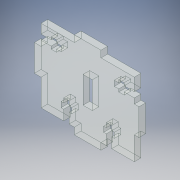
# Autodesk Inventor part: Refuerzo_Conducto
Saved by Autodesk Inventor 2019 (Build 230136000, 136)
## iProperties
Created: 2020-04-06
Part Number: Refuerzo_Conducto
Material: Generic
Document SubType Name: Modeling
Designer: Jurgen
Density: 1 g/cm^3
Appearance: Clear
Author: Jurgen
Autodesk Inventor part; units mm, degrees
ref_plane "YZ Plane" through (0, 0, 0) normal (1, 0, 0) x (0, 1, 0)
ref_plane "XZ Plane" through (0, 0, 0) normal (0, 1, 0) x (-1, 0, 0)
ref_plane "XY Plane" through (0, 0, 0) normal (0, 0, 1) x (1, 0, 0)
sketch "Sketch1" plane through (0, 0, 0) normal (0, 0, 1) x (1, 0, 0)
  line L0 (-35, -27.5) -> (35, -27.5)
  line L1 (35, -27.5) -> (35, 27.5)
  line L2 (35, 27.5) -> (-35, 27.5)
  line L3 (-35, 27.5) -> (-35, -27.5)
  line L4 (-35, -27.5) -> (35, 27.5) construction
  line L5 (35, -27.5) -> (-35, 27.5) construction
  point P0 (0, 0)
  dimension "d0" = 70
  dimension "d1" = 55
  constraints: 12 end point, 2 midpoint, 2 parallel, 1 horizontal, 1 perpendicular
  measures "d0" distance of L2.end L1.end
  measures "d1" distance of L1.end L0.end
extrude "Extrusion1" add sketch "Sketch1" along normal blind 5
sketch "Sketch2" plane through (0, 0, 5) normal (0, 0, 1) x (1, 0, 0)
  line L0 (-35, -27.5) -> (35, -27.5) construction
  line L1 (35, -27.5) -> (35, 27.5) construction
  line L2 (35, 27.5) -> (-35, 27.5) construction
  line L3 (-35, 27.5) -> (-35, -27.5) construction
  line L4 (-10, -27.5) -> (10, -27.5)
  line L5 (10, -27.5) -> (10, -32.5)
  line L6 (10, -32.5) -> (-10, -32.5)
  line L7 (-10, -32.5) -> (-10, -27.5)
  line L8 (-35, -7.5) -> (-40, -7.5)
  line L9 (-40, -7.5) -> (-40, 12.5)
  line L10 (-40, 12.5) -> (-35, 12.5)
  line L11 (-35, 12.5) -> (-35, -7.5)
  line L12 (35, 27.5) -> (-35, 27.5) construction
  line L13 (-10, 27.5) -> (10, 27.5)
  line L14 (10, 27.5) -> (10, 32.5)
  line L15 (10, 32.5) -> (-10, 32.5)
  line L16 (-10, 32.5) -> (-10, 27.5)
  line L17 (35, 18) -> (35, 14) construction
  line L18 (35, 14) -> (20, 14) construction
  line L19 (20, 14) -> (20, 18) construction
  line L20 (20, 18) -> (35, 18) construction
  line L21 (35, 16) -> (20, 16) construction
  line L22 (23.3333, 20) -> (23.3333, 12) construction
  line L23 (23.3333, 12) -> (27.3333, 12) construction
  line L24 (27.3333, 12) -> (27.3333, 20) construction
  line L25 (27.3333, 20) -> (23.3333, 20) construction
  line L26 (23.3333, 20) -> (27.3333, 12) construction
  line L27 (23.3333, 12) -> (27.3333, 20) construction
  line L28 (35, 18) -> (27.3333, 18)
  line L29 (27.3333, 18) -> (27.3333, 20)
  line L30 (27.3333, 20) -> (23.3333, 20)
  line L31 (23.3333, 20) -> (23.3333, 18)
  line L32 (23.3333, 18) -> (20, 18)
  line L33 (20, 18) -> (20, 14)
  line L34 (20, 14) -> (23.3333, 14)
  line L35 (23.3333, 14) -> (23.3333, 12)
  line L36 (23.3333, 12) -> (27.3333, 12)
  line L37 (27.3333, 12) -> (27.3333, 14)
  line L38 (27.3333, 14) -> (35, 14)
  line L39 (35, 14) -> (35, 18)
  line L40 (-35, 16.5) -> (-35, 20.5) construction
  line L41 (-35, 20.5) -> (-20, 20.5) construction
  line L42 (-20, 20.5) -> (-20, 16.5) construction
  line L43 (-20, 16.5) -> (-35, 16.5) construction
  line L44 (-35, 18.5) -> (-20, 18.5) construction
  line L45 (-23.3333, 14.5) -> (-23.3333, 22.5) construction
  line L46 (-23.3333, 22.5) -> (-27.3333, 22.5) construction
  line L47 (-27.3333, 22.5) -> (-27.3333, 14.5) construction
  line L48 (-27.3333, 14.5) -> (-23.3333, 14.5) construction
  line L49 (-23.3333, 14.5) -> (-27.3333, 22.5) construction
  line L50 (-23.3333, 22.5) -> (-27.3333, 14.5) construction
  line L51 (-35, 16.5) -> (-27.3333, 16.5)
  line L52 (-27.3333, 16.5) -> (-27.3333, 14.5)
  line L53 (-27.3333, 14.5) -> (-23.3333, 14.5)
  line L54 (-23.3333, 14.5) -> (-23.3333, 16.5)
  line L55 (-23.3333, 16.5) -> (-20, 16.5)
  line L56 (-20, 16.5) -> (-20, 20.5)
  line L57 (-20, 20.5) -> (-23.3333, 20.5)
  line L58 (-23.3333, 20.5) -> (-23.3333, 22.5)
  line L59 (-23.3333, 22.5) -> (-27.3333, 22.5)
  line L60 (-27.3333, 22.5) -> (-27.3333, 20.5)
  line L61 (-27.3333, 20.5) -> (-35, 20.5)
  line L62 (-35, 20.5) -> (-35, 16.5)
  line L63 (-14, -27.5) -> (-18, -27.5) construction
  line L64 (-18, -27.5) -> (-18, -12.5) construction
  line L65 (-18, -12.5) -> (-14, -12.5) construction
  line L66 (-14, -12.5) -> (-14, -27.5) construction
  line L67 (-16, -27.5) -> (-16, -12.5) construction
  line L68 (-12, -15.8333) -> (-20, -15.8333) construction
  line L69 (-20, -15.8333) -> (-20, -19.8333) construction
  line L70 (-20, -19.8333) -> (-12, -19.8333) construction
  line L71 (-12, -19.8333) -> (-12, -15.8333) construction
  line L72 (-12, -15.8333) -> (-20, -19.8333) construction
  line L73 (-20, -15.8333) -> (-12, -19.8333) construction
  line L74 (-14, -27.5) -> (-14, -19.8333)
  line L75 (-14, -19.8333) -> (-12, -19.8333)
  line L76 (-12, -19.8333) -> (-12, -15.8333)
  line L77 (-12, -15.8333) -> (-14, -15.8333)
  line L78 (-14, -15.8333) -> (-14, -12.5)
  line L79 (-14, -12.5) -> (-18, -12.5)
  line L80 (-18, -12.5) -> (-18, -15.8333)
  line L81 (-18, -15.8333) -> (-20, -15.8333)
  line L82 (-20, -15.8333) -> (-20, -19.8333)
  line L83 (-20, -19.8333) -> (-18, -19.8333)
  line L84 (-18, -19.8333) -> (-18, -27.5)
  line L85 (-18, -27.5) -> (-14, -27.5)
  line L86 (18, -27.5) -> (14, -27.5) construction
  line L87 (14, -27.5) -> (14, -12.5) construction
  line L88 (14, -12.5) -> (18, -12.5) construction
  line L89 (18, -12.5) -> (18, -27.5) construction
  line L90 (16, -27.5) -> (16, -12.5) construction
  line L91 (20, -15.8333) -> (12, -15.8333) construction
  line L92 (12, -15.8333) -> (12, -19.8333) construction
  line L93 (12, -19.8333) -> (20, -19.8333) construction
  line L94 (20, -19.8333) -> (20, -15.8333) construction
  line L95 (20, -15.8333) -> (12, -19.8333) construction
  line L96 (12, -15.8333) -> (20, -19.8333) construction
  line L97 (18, -27.5) -> (18, -19.8333)
  line L98 (18, -19.8333) -> (20, -19.8333)
  line L99 (20, -19.8333) -> (20, -15.8333)
  line L100 (20, -15.8333) -> (18, -15.8333)
  line L101 (18, -15.8333) -> (18, -12.5)
  line L102 (18, -12.5) -> (14, -12.5)
  line L103 (14, -12.5) -> (14, -15.8333)
  line L104 (14, -15.8333) -> (12, -15.8333)
  line L105 (12, -15.8333) -> (12, -19.8333)
  line L106 (12, -19.8333) -> (14, -19.8333)
  line L107 (14, -19.8333) -> (14, -27.5)
  line L108 (14, -27.5) -> (18, -27.5)
  line L109 (35, -27.5) -> (35, 27.5) construction
  line L110 (35, 10) -> (38.5, 10)
  line L111 (38.5, 10) -> (38.5, -10)
  line L112 (38.5, -10) -> (35, -10)
  line L113 (35, -10) -> (35, 10)
  point P0 (0, 0)
  point P1 (25.3333, 16)
  point P2 (-25.3333, 18.5)
  point P3 (-16, -17.8333)
  point P4 (16, -17.8333)
  dimension "d4" = 20
  dimension "d5" = 5
  dimension "d6" = 25
  dimension "d7" = 5
  dimension "d8" = 20
  dimension "d9" = 20
  dimension "d10" = 20
  dimension "d11" = 5
  dimension "d12" = 25
  dimension "d13" = 4
  dimension "d14" = 15
  dimension "d15" = 8
  dimension "d16" = 4
  dimension "d22" = 4
  dimension "d23" = 15
  dimension "d24" = 8
  dimension "d25" = 4
  dimension "d26" = 4
  dimension "d28" = 4
  dimension "d29" = 15
  dimension "d30" = 8
  dimension "d31" = 4
  dimension "d32" = 4
  dimension "d33" = 15
  dimension "d34" = 8
  dimension "d35" = 4
  dimension "d36" = 8
  dimension "d37" = 4
  dimension "d38" = 3.5
  dimension "d39" = 20
  dimension "d40" = 17.5
  dimension "d41" = 4
  constraints: 216 end point, 44 point on line, 32 perpendicular, 24 parallel, 16 midpoint, 4 collinear, 4 horizontal
  measures "d4" distance of L5.end L6.end
  measures "d5" distance of L4.end L5.end
  measures "d6" distance between parallel lines of L3 L7
  measures "d7" distance of L9.end L10.end
  measures "d8" distance of L8.end L9.end
  measures "d9" distance between parallel lines of L0 L8
  measures "d10" distance of L15.end L14.end
  measures "d11" distance of L14.end L13.end
  measures "d12" distance between parallel lines of L3 L16
  measures "d13" distance of L18.end L19.end
  measures "d14" distance of L17.end L18.end
  measures "d15" distance of L24.end L23.end
  measures "d16" distance of L23.end L22.end
  measures "d22" distance of L41.end L55.end
  measures "d23" distance of L40.end L41.end
  measures "d24" distance of L48.start L47.start
  measures "d25" distance of L47.start L45.end
  measures "d26" distance between parallel lines of L10 L43
  measures "d28" distance of L64.end L66.start
  measures "d29" distance of L63.end L64.end
  measures "d30" distance of L70.end L70.start
  measures "d31" distance of L70.start L73.start
  measures "d32" distance of L87.end L89.start
  measures "d33" distance of L86.end L87.end
  measures "d34" distance of L93.end L93.start
  measures "d35" distance of L93.start L96.start
  measures "d36" distance between parallel lines of L64 L7
  measures "d37" distance between parallel lines of L5 L107
  measures "d38" distance of L111.end L112.end
  measures "d39" distance of L110.end L111.end
  measures "d40" distance between parallel lines of L110 L2
  measures "d41" distance between parallel lines of L110 L38
extrude "Extrusion2" add sketch "Sketch2" against normal blind 5 contours L4 L5 L6 L7 | L8 L9 L10 L11 | L16 L15 L14 L13 | L110 L111 L112 L113
sketch "Sketch3" plane through (0, 0, 5) normal (0, 0, 1) x (1, 0, 0)
  line L0 (-35, -27.5) -> (35, -27.5) construction
  line L1 (35, -27.5) -> (35, 27.5) construction
  line L2 (35, 27.5) -> (-35, 27.5) construction
  line L3 (-35, 27.5) -> (-35, -27.5) construction
  line L4 (-10, -27.5) -> (10, -27.5)
  line L5 (10, -27.5) -> (10, -32.5)
  line L6 (10, -32.5) -> (-10, -32.5)
  line L7 (-10, -32.5) -> (-10, -27.5)
  line L8 (-35, -7.5) -> (-40, -7.5)
  line L9 (-40, -7.5) -> (-40, 12.5)
  line L10 (-40, 12.5) -> (-35, 12.5)
  line L11 (-35, 12.5) -> (-35, -7.5)
  line L12 (35, 27.5) -> (-35, 27.5) construction
  line L13 (-15, 27.5) -> (10, 27.5)
  line L14 (10, 27.5) -> (10, 32.5)
  line L15 (10, 32.5) -> (-15, 32.5)
  line L16 (-15, 32.5) -> (-15, 27.5)
  line L17 (35, 18) -> (35, 14) construction
  line L18 (35, 14) -> (20, 14) construction
  line L19 (20, 14) -> (20, 18) construction
  line L20 (20, 18) -> (35, 18) construction
  line L21 (35, 16) -> (20, 16) construction
  line L22 (23.3333, 20) -> (23.3333, 12) construction
  line L23 (23.3333, 12) -> (27.3333, 12) construction
  line L24 (27.3333, 12) -> (27.3333, 20) construction
  line L25 (27.3333, 20) -> (23.3333, 20) construction
  line L26 (23.3333, 20) -> (27.3333, 12) construction
  line L27 (23.3333, 12) -> (27.3333, 20) construction
  line L28 (35, 18) -> (27.3333, 18)
  line L29 (27.3333, 18) -> (27.3333, 20)
  line L30 (27.3333, 20) -> (23.3333, 20)
  line L31 (23.3333, 20) -> (23.3333, 18)
  line L32 (23.3333, 18) -> (20, 18)
  line L33 (20, 18) -> (20, 14)
  line L34 (20, 14) -> (23.3333, 14)
  line L35 (23.3333, 14) -> (23.3333, 12)
  line L36 (23.3333, 12) -> (27.3333, 12)
  line L37 (27.3333, 12) -> (27.3333, 14)
  line L38 (27.3333, 14) -> (35, 14)
  line L39 (35, 14) -> (35, 18)
  line L40 (-27.3333, 14.5) -> (-23.3333, 14.5) construction
  line L41 (-27.3333, 14.5) -> (-23.3333, 14.5)
  line L42 (-23.3333, 14.5) -> (-23.3333, 16.5)
  line L43 (-27.3333, 22.5) -> (-27.3333, 14.5) construction
  line L44 (-23.3333, 14.5) -> (-23.3333, 22.5) construction
  line L45 (-23.3333, 14.5) -> (-27.3333, 22.5) construction
  line L46 (-23.3333, 22.5) -> (-27.3333, 14.5) construction
  line L47 (-23.3333, 16.5) -> (-20, 16.5)
  line L48 (-35, 16.5) -> (-27.3333, 16.5)
  line L49 (-27.3333, 22.5) -> (-27.3333, 20.5)
  line L50 (-23.3333, 20.5) -> (-23.3333, 22.5)
  line L51 (-23.3333, 22.5) -> (-27.3333, 22.5) construction
  line L52 (-23.3333, 22.5) -> (-27.3333, 22.5)
  line L53 (-35, 16.5) -> (-35, 20.5) construction
  line L54 (-35, 20.5) -> (-35, 16.5)
  line L55 (-27.3333, 20.5) -> (-35, 20.5)
  line L56 (-20, 16.5) -> (-35, 16.5) construction
  line L57 (-35, 18.5) -> (-20, 18.5) construction
  line L58 (-35, 20.5) -> (-20, 20.5) construction
  line L59 (-27.3333, 16.5) -> (-27.3333, 14.5)
  line L60 (-20, 20.5) -> (-20, 16.5) construction
  line L61 (-20, 16.5) -> (-20, 20.5)
  line L62 (-20, 20.5) -> (-23.3333, 20.5)
  line L63 (-14, -27.5) -> (-18, -27.5) construction
  line L64 (-18, -27.5) -> (-18, -12.5) construction
  line L65 (-14, -12.5) -> (-14, -27.5) construction
  line L66 (-16, -27.5) -> (-16, -12.5) construction
  line L67 (-18, -19.8333) -> (-18, -27.5)
  line L68 (-14, -27.5) -> (-14, -19.8333)
  line L69 (-18, -27.5) -> (-14, -27.5)
  line L70 (-20, -19.8333) -> (-12, -19.8333) construction
  line L71 (-20, -19.8333) -> (-18, -19.8333)
  line L72 (-14, -19.8333) -> (-12, -19.8333)
  line L73 (-12, -15.8333) -> (-20, -19.8333) construction
  line L74 (-12, -19.8333) -> (-12, -15.8333) construction
  line L75 (-12, -19.8333) -> (-12, -15.8333)
  line L76 (-20, -15.8333) -> (-12, -19.8333) construction
  line L77 (-12, -15.8333) -> (-14, -15.8333)
  line L78 (-12, -15.8333) -> (-20, -15.8333) construction
  line L79 (-20, -15.8333) -> (-20, -19.8333)
  line L80 (-18, -15.8333) -> (-20, -15.8333)
  line L81 (-14, -15.8333) -> (-14, -12.5)
  line L82 (-18, -12.5) -> (-14, -12.5) construction
  line L83 (-14, -12.5) -> (-18, -12.5)
  line L84 (-18, -12.5) -> (-18, -15.8333)
  line L85 (-20, -15.8333) -> (-20, -19.8333) construction
  line L86 (18, -27.5) -> (14, -27.5) construction
  line L87 (14, -27.5) -> (14, -12.5) construction
  line L88 (18, -12.5) -> (18, -27.5) construction
  line L89 (16, -27.5) -> (16, -12.5) construction
  line L90 (14, -19.8333) -> (14, -27.5)
  line L91 (18, -27.5) -> (18, -19.8333)
  line L92 (14, -27.5) -> (18, -27.5)
  line L93 (12, -19.8333) -> (20, -19.8333) construction
  line L94 (12, -19.8333) -> (14, -19.8333)
  line L95 (18, -19.8333) -> (20, -19.8333)
  line L96 (20, -15.8333) -> (12, -19.8333) construction
  line L97 (20, -19.8333) -> (20, -15.8333) construction
  line L98 (20, -19.8333) -> (20, -15.8333)
  line L99 (12, -15.8333) -> (20, -19.8333) construction
  line L100 (20, -15.8333) -> (18, -15.8333)
  line L101 (20, -15.8333) -> (12, -15.8333) construction
  line L102 (12, -15.8333) -> (12, -19.8333)
  line L103 (14, -15.8333) -> (12, -15.8333)
  line L104 (18, -15.8333) -> (18, -12.5)
  line L105 (14, -12.5) -> (18, -12.5) construction
  line L106 (18, -12.5) -> (14, -12.5)
  line L107 (14, -12.5) -> (14, -15.8333)
  line L108 (12, -15.8333) -> (12, -19.8333) construction
  line L109 (35, -27.5) -> (35, 27.5) construction
  line L110 (35, 10) -> (40, 10)
  line L111 (40, 10) -> (40, -10)
  line L112 (40, -10) -> (35, -10)
  line L113 (35, -10) -> (35, 10)
  point P0 (0, 0)
  point P1 (0, 0)
  point P2 (25.3333, 16)
  point P3 (-25.3333, 18.5)
  point P4 (-16, -17.8333)
  point P5 (16, -17.8333)
  dimension "d44" = 20
  dimension "d45" = 5
  dimension "d46" = 25
  dimension "d47" = 5
  dimension "d48" = 20
  dimension "d49" = 20
  dimension "d50" = 25
  dimension "d51" = 5
  dimension "d52" = 20
  dimension "d53" = 4
  dimension "d54" = 15
  dimension "d55" = 8
  dimension "d56" = 4
  dimension "d57" = 4
  dimension "d58" = 15
  dimension "d59" = 8
  dimension "d60" = 4
  dimension "d61" = 4
  dimension "d62" = 4
  dimension "d63" = 15
  dimension "d64" = 8
  dimension "d65" = 4
  dimension "d66" = 4
  dimension "d67" = 15
  dimension "d68" = 8
  dimension "d69" = 4
  dimension "d70" = 8
  dimension "d71" = 4
  dimension "d72" = 5
  dimension "d73" = 20
  dimension "d74" = 17.5
  dimension "d75" = 4
  constraints: 228 end point, 44 point on line, 32 perpendicular, 24 parallel, 16 midpoint, 4 collinear, 4 horizontal
  measures "d44" distance of L5.end L6.end
  measures "d45" distance of L4.end L5.end
  measures "d46" distance between parallel lines of L3 L7
  measures "d47" distance of L9.end L10.end
  measures "d48" distance of L8.end L9.end
  measures "d49" distance between parallel lines of L0 L8
  measures "d50" distance of L15.end L14.end
  measures "d51" distance of L14.end L13.end
  measures "d52" distance between parallel lines of L3 L16
  measures "d53" distance of L18.end L19.end
  measures "d54" distance of L17.end L18.end
  measures "d55" distance of L24.end L23.end
  measures "d56" distance of L23.end L22.end
  measures "d57" distance of L58.end L47.end
  measures "d58" distance of L53.end L58.end
  measures "d59" distance of L40.start L43.start
  measures "d60" distance of L43.start L44.end
  measures "d61" distance between parallel lines of L10 L56
  measures "d62" distance of L64.end L65.start
  measures "d63" distance of L63.end L64.end
  measures "d64" distance of L70.end L70.start
  measures "d65" distance of L70.start L76.start
  measures "d66" distance of L87.end L88.start
  measures "d67" distance of L86.end L87.end
  measures "d68" distance of L93.end L93.start
  measures "d69" distance of L93.start L99.start
  measures "d70" distance between parallel lines of L64 L7
  measures "d71" distance between parallel lines of L5 L90
  measures "d72" distance of L111.end L112.end
  measures "d73" distance of L110.end L111.end
  measures "d74" distance between parallel lines of L110 L2
  measures "d75" distance between parallel lines of L110 L38
extrude "Extrusion3" cut sketch "Sketch3" against normal blind 5 contours L39 L38 L37 L36 L35 L34 L33 L32 L31 L30 L29 L28 | L59 L48 L54 L55 L49 L52 L50 L62 L61 L47 L42 L41 | L71 L79 L80 L84 L83 L81 L77 L75 L72 L68 L69 L67 | L94 L102 L103 L107 L106 L104 L100 L98 L95 L91 L92 L90
sketch "Sketch4" plane through (0, 0, 5) normal (0, 0, 1) x (1, 0, 0)
  line L0 (-14, -19.8333) -> (-14, -27.5) construction
  line L1 (-14, -27.5) -> (-10, -27.5) construction
  line L2 (-10, -32.5) -> (-10, -27.5) construction
  line L3 (10, -32.5) -> (-10, -32.5) construction
  line L4 (10, -27.5) -> (10, -32.5) construction
  line L5 (10, -27.5) -> (14, -27.5) construction
  line L6 (14, -27.5) -> (14, -19.8333) construction
  line L7 (14, -19.8333) -> (12, -19.8333) construction
  line L8 (12, -19.8333) -> (12, -15.8333) construction
  line L9 (12, -15.8333) -> (14, -15.8333) construction
  line L10 (14, -15.8333) -> (14, -12.5) construction
  line L11 (14, -12.5) -> (18, -12.5) construction
  line L12 (18, -12.5) -> (18, -15.8333) construction
  line L13 (18, -15.8333) -> (20, -15.8333) construction
  line L14 (20, -15.8333) -> (20, -19.8333) construction
  line L15 (20, -19.8333) -> (18, -19.8333) construction
  line L16 (18, -19.8333) -> (18, -27.5) construction
  line L17 (18, -27.5) -> (35, -27.5) construction
  line L18 (35, -27.5) -> (35, -10) construction
  line L19 (38.5, -10) -> (35, -10) construction
  line L20 (38.5, 10) -> (38.5, -10) construction
  line L21 (35, 10) -> (38.5, 10) construction
  line L22 (35, 10) -> (35, 14) construction
  line L23 (35, 14) -> (27.3333, 14) construction
  line L24 (27.3333, 14) -> (27.3333, 12) construction
  line L25 (27.3333, 12) -> (23.3333, 12) construction
  line L26 (23.3333, 12) -> (23.3333, 14) construction
  line L27 (23.3333, 14) -> (20, 14) construction
  line L28 (20, 14) -> (20, 18) construction
  line L29 (20, 18) -> (23.3333, 18) construction
  line L30 (23.3333, 18) -> (23.3333, 20) construction
  line L31 (23.3333, 20) -> (27.3333, 20) construction
  line L32 (27.3333, 20) -> (27.3333, 18) construction
  line L33 (27.3333, 18) -> (35, 18) construction
  line L34 (35, 18) -> (35, 27.5) construction
  line L35 (35, 27.5) -> (10, 27.5) construction
  line L36 (10, 27.5) -> (10, 32.5) construction
  line L37 (10, 32.5) -> (-10, 32.5) construction
  line L38 (-10, 32.5) -> (-10, 27.5) construction
  line L39 (-10, 27.5) -> (-35, 27.5) construction
  line L40 (-35, 27.5) -> (-35, 20.5) construction
  line L41 (-35, 20.5) -> (-27.3333, 20.5) construction
  line L42 (-27.3333, 20.5) -> (-27.3333, 22.5) construction
  line L43 (-27.3333, 22.5) -> (-23.3333, 22.5) construction
  line L44 (-23.3333, 22.5) -> (-23.3333, 20.5) construction
  line L45 (-23.3333, 20.5) -> (-20, 20.5) construction
  line L46 (-20, 20.5) -> (-20, 16.5) construction
  line L47 (-20, 16.5) -> (-23.3333, 16.5) construction
  line L48 (-23.3333, 16.5) -> (-23.3333, 14.5) construction
  line L49 (-23.3333, 14.5) -> (-27.3333, 14.5) construction
  line L50 (-27.3333, 14.5) -> (-27.3333, 16.5) construction
  line L51 (-27.3333, 16.5) -> (-35, 16.5) construction
  line L52 (-35, 16.5) -> (-35, 12.5) construction
  line L53 (-40, 12.5) -> (-35, 12.5) construction
  line L54 (-40, -7.5) -> (-40, 12.5) construction
  line L55 (-35, -7.5) -> (-40, -7.5) construction
  line L56 (-35, -7.5) -> (-35, -27.5) construction
  line L57 (-35, -27.5) -> (-18, -27.5) construction
  line L58 (-18, -27.5) -> (-18, -19.8333) construction
  line L59 (-18, -19.8333) -> (-20, -19.8333) construction
  line L60 (-20, -19.8333) -> (-20, -15.8333) construction
  line L61 (-20, -15.8333) -> (-18, -15.8333) construction
  line L62 (-18, -15.8333) -> (-18, -12.5) construction
  line L63 (-18, -12.5) -> (-14, -12.5) construction
  line L64 (-14, -12.5) -> (-14, -15.8333) construction
  line L65 (-14, -15.8333) -> (-12, -15.8333) construction
  line L66 (-12, -15.8333) -> (-12, -19.8333) construction
  line L67 (-12, -19.8333) -> (-14, -19.8333) construction
  line L68 (0, 32.5) -> (0, -32.5) construction
  line L69 (-40, 0) -> (38.5, 0) construction
  line L70 (-3.5, -10) -> (3.5, -10)
  line L71 (3.5, -10) -> (3.5, 10)
  line L72 (3.5, 10) -> (-3.5, 10)
  line L73 (-3.5, 10) -> (-3.5, -10)
  line L74 (-3.5, -10) -> (3.5, 10) construction
  line L75 (3.5, -10) -> (-3.5, 10) construction
  point P0 (0, 0)
  dimension "d80" = 7
  dimension "d81" = 20
  constraints: 16 end point, 5 midpoint, 2 parallel, 1 horizontal, 1 perpendicular, 1 point on line
  measures "d80" distance of L72.end L71.end
  measures "d81" distance of L71.end L70.end
extrude "Extrusion4" cut sketch "Sketch4" against normal blind 10
body "Solid1"
